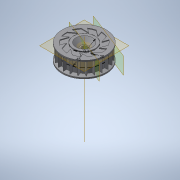
# Autodesk Inventor part: rear-wheel
Saved by Autodesk Inventor 2020 (Build 240168000, 168)
## iProperties
Created: 2020-01-27
Part Number: rear-wheel
Material: Ogólne
Document SubType Name: Modeling
Designer: blep
Density: 1 g/cm^3
Appearance: Domyślne
Author: blep
Autodesk Inventor part; units mm, degrees
ref_plane "YZ Plane" through (0, 0, 0) normal (1, 0, 0) x (0, 1, 0)
ref_plane "XZ Plane" through (0, 0, 0) normal (0, 1, 0) x (-1, 0, 0)
ref_plane "XY Plane" through (0, 0, 0) normal (0, 0, 1) x (1, 0, 0)
sketch "Sketch1" plane through (0, 0, 0) normal (0, 0, 1) x (1, 0, 0)
  line L0 (0.8361, -0.5831) -> (0.755, -0.1219) projected
  line L1 (0.6595, -0.0924) -> (0.3327, -0.4279) projected
  arc A0 (0.755, -0.1219) -> (0.6595, -0.0924) centre (0, -2.4) ccw projected
  arc A1 (0.3327, -0.4279) -> (0.2337, -0.4137) centre (0, -2.4) ccw projected
  arc A2 (0.9258, -0.6272) -> (0.8361, -0.5831) centre (0, -2.4) ccw projected
  line L2 (1.3403, -0.4091) -> (0.9258, -0.6272) projected
  arc A3 (1.4221, -0.4667) -> (1.3403, -0.4091) centre (0, -2.4) ccw projected
  line L3 (1.3566, -0.9304) -> (1.4221, -0.4667) projected
  arc A4 (1.4283, -1.0001) -> (1.3566, -0.9304) centre (0, -2.4) ccw projected
  line L4 (1.8899, -0.9207) -> (1.4283, -1.0001) projected
  arc A5 (1.9499, -1.0007) -> (1.8899, -0.9207) centre (0, -2.4) ccw projected
  line L5 (1.7443, -1.4216) -> (1.9499, -1.0007) projected
  arc A6 (1.791, -1.51) -> (1.7443, -1.4216) centre (0, -2.4) ccw projected
  line L6 (2.2545, -1.5772) -> (1.791, -1.51) projected
  arc A7 (2.2869, -1.6718) -> (2.2545, -1.5772) centre (0, -2.4) ccw projected
  line L7 (1.9613, -2.0085) -> (2.2869, -1.6718) projected
  arc A8 (1.9784, -2.107) -> (1.9613, -2.0085) centre (0, -2.4) ccw projected
  line L8 (2.3985, -2.3141) -> (1.9784, -2.107) projected
  arc A9 (2.4, -2.4141) -> (2.3985, -2.3141) centre (0, -2.4) ccw projected
  line L9 (1.9863, -2.6337) -> (2.4, -2.4141) projected
  arc A10 (1.9721, -2.7327) -> (1.9863, -2.6337) centre (0, -2.4) ccw projected
  line L10 (2.3076, -3.0595) -> (1.9721, -2.7327) projected
  line L11 (1.8169, -3.2361) -> (2.2781, -3.155) projected
  arc A11 (2.2781, -3.155) -> (2.3076, -3.0595) centre (0, -2.4) ccw projected
  arc A12 (1.7728, -3.3258) -> (1.8169, -3.2361) centre (0, -2.4) ccw projected
  line L12 (1.9909, -3.7403) -> (1.7728, -3.3258) projected
  arc A13 (1.9333, -3.8221) -> (1.9909, -3.7403) centre (0, -2.4) ccw projected
  line L13 (1.4696, -3.7566) -> (1.9333, -3.8221) projected
  arc A14 (1.3999, -3.8283) -> (1.4696, -3.7566) centre (0, -2.4) ccw projected
  line L14 (1.4793, -4.2899) -> (1.3999, -3.8283) projected
  arc A15 (1.3993, -4.3499) -> (1.4793, -4.2899) centre (0, -2.4) ccw projected
  line L15 (0.9784, -4.1443) -> (1.3993, -4.3499) projected
  arc A16 (0.89, -4.191) -> (0.9784, -4.1443) centre (0, -2.4) ccw projected
  line L16 (0.8228, -4.6545) -> (0.89, -4.191) projected
  arc A17 (0.7282, -4.6869) -> (0.8228, -4.6545) centre (0, -2.4) ccw projected
  line L17 (0.3915, -4.3613) -> (0.7282, -4.6869) projected
  arc A18 (0.293, -4.3784) -> (0.3915, -4.3613) centre (0, -2.4) ccw projected
  line L18 (0.0859, -4.7985) -> (0.293, -4.3784) projected
  arc A19 (-0.0141, -4.8) -> (0.0859, -4.7985) centre (0, -2.4) ccw projected
  line L19 (-0.2337, -4.3863) -> (-0.0141, -4.8) projected
  arc A20 (-0.3327, -4.3721) -> (-0.2337, -4.3863) centre (0, -2.4) ccw projected
  line L20 (-0.6595, -4.7076) -> (-0.3327, -4.3721) projected
  arc A21 (-0.755, -4.6781) -> (-0.6595, -4.7076) centre (0, -2.4) ccw projected
  line L21 (-0.8361, -4.2169) -> (-0.755, -4.6781) projected
  arc A22 (-0.9258, -4.1728) -> (-0.8361, -4.2169) centre (0, -2.4) ccw projected
  line L22 (-1.3403, -4.3909) -> (-0.9258, -4.1728) projected
  arc A23 (-1.4221, -4.3333) -> (-1.3403, -4.3909) centre (0, -2.4) ccw projected
  line L23 (-1.3566, -3.8696) -> (-1.4221, -4.3333) projected
  arc A24 (-1.4283, -3.7999) -> (-1.3566, -3.8696) centre (0, -2.4) ccw projected
  line L24 (-1.8899, -3.8793) -> (-1.4283, -3.7999) projected
  arc A25 (-1.9499, -3.7993) -> (-1.8899, -3.8793) centre (0, -2.4) ccw projected
  line L25 (-1.7443, -3.3784) -> (-1.9499, -3.7993) projected
  arc A26 (-1.791, -3.29) -> (-1.7443, -3.3784) centre (0, -2.4) ccw projected
  line L26 (-2.2545, -3.2228) -> (-1.791, -3.29) projected
  arc A27 (-2.2869, -3.1282) -> (-2.2545, -3.2228) centre (0, -2.4) ccw projected
  line L27 (-1.9613, -2.7915) -> (-2.2869, -3.1282) projected
  arc A28 (-1.9784, -2.693) -> (-1.9613, -2.7915) centre (0, -2.4) ccw projected
  line L28 (-2.3985, -2.4859) -> (-1.9784, -2.693) projected
  arc A29 (-2.4, -2.3859) -> (-2.3985, -2.4859) centre (0, -2.4) ccw projected
  line L29 (-1.9863, -2.1663) -> (-2.4, -2.3859) projected
  arc A30 (-1.9721, -2.0673) -> (-1.9863, -2.1663) centre (0, -2.4) ccw projected
  line L30 (-2.3076, -1.7405) -> (-1.9721, -2.0673) projected
  arc A31 (-2.2781, -1.645) -> (-2.3076, -1.7405) centre (0, -2.4) ccw projected
  line L31 (-1.8169, -1.5639) -> (-2.2781, -1.645) projected
  arc A32 (-1.7728, -1.4742) -> (-1.8169, -1.5639) centre (0, -2.4) ccw projected
  line L32 (-1.9909, -1.0597) -> (-1.7728, -1.4742) projected
  arc A33 (-1.9333, -0.9779) -> (-1.9909, -1.0597) centre (0, -2.4) ccw projected
  line L33 (-1.4696, -1.0434) -> (-1.9333, -0.9779) projected
  arc A34 (-1.3999, -0.9717) -> (-1.4696, -1.0434) centre (0, -2.4) ccw projected
  line L34 (-1.4793, -0.5101) -> (-1.3999, -0.9717) projected
  arc A35 (-1.3993, -0.4501) -> (-1.4793, -0.5101) centre (0, -2.4) ccw projected
  line L35 (-0.9784, -0.6557) -> (-1.3993, -0.4501) projected
  arc A36 (-0.89, -0.609) -> (-0.9784, -0.6557) centre (0, -2.4) ccw projected
  line L36 (-0.8228, -0.1455) -> (-0.89, -0.609) projected
  arc A37 (-0.7282, -0.1131) -> (-0.8228, -0.1455) centre (0, -2.4) ccw projected
  line L37 (-0.3915, -0.4387) -> (-0.7282, -0.1131) projected
  arc A38 (-0.293, -0.4216) -> (-0.3915, -0.4387) centre (0, -2.4) ccw projected
  line L38 (-0.0859, -0.0015) -> (-0.293, -0.4216) projected
  arc A39 (0.0141, 0) -> (-0.0859, -0.0015) centre (0, -2.4) ccw projected
  line L39 (0.2337, -0.4137) -> (0.0141, 0) projected
  line L40 (-0.4177, 0.0039) -> (-0.6435, 0.2222)
  arc A40 (-0.6435, 0.2222) -> (-1.095, 0.068) centre (0, -2.4) ccw
  line L41 (-1.095, 0.068) -> (-1.1401, -0.2428)
  line L42 (-1.1401, -0.2428) -> (-1.4223, -0.105)
  arc A41 (-1.4223, -0.105) -> (-1.8041, -0.3912) centre (0, -2.4) ccw
  line L43 (-1.8041, -0.3912) -> (-1.7509, -0.7007)
  line L44 (-1.7509, -0.7007) -> (-2.0619, -0.6568)
  arc A42 (-2.0619, -0.6568) -> (-2.3365, -1.047) centre (0, -2.4) ccw
  line L45 (-2.3365, -1.047) -> (-2.1903, -1.3249)
  line L46 (-2.1903, -1.3249) -> (-2.4996, -1.3793)
  arc A43 (-2.4996, -1.3793) -> (-2.6403, -1.8353) centre (0, -2.4) ccw
  line L47 (-2.6403, -1.8353) -> (-2.4153, -2.0544)
  line L48 (-2.4153, -2.0544) -> (-2.6927, -2.2017)
  arc A44 (-2.6927, -2.2017) -> (-2.6856, -2.6788) centre (0, -2.4) ccw
  line L49 (-2.6856, -2.6788) -> (-2.4039, -2.8177)
  line L50 (-2.4039, -2.8177) -> (-2.6222, -3.0435)
  arc A45 (-2.6222, -3.0435) -> (-2.468, -3.495) centre (0, -2.4) ccw
  line L51 (-2.468, -3.495) -> (-2.1572, -3.5401)
  line L52 (-2.1572, -3.5401) -> (-2.295, -3.8223)
  arc A46 (-2.295, -3.8223) -> (-2.0088, -4.2041) centre (0, -2.4) ccw
  line L53 (-2.0088, -4.2041) -> (-1.6993, -4.1509)
  line L54 (-1.6993, -4.1509) -> (-1.7432, -4.4619)
  arc A47 (-1.7432, -4.4619) -> (-1.353, -4.7365) centre (0, -2.4) ccw
  line L55 (-1.353, -4.7365) -> (-1.0751, -4.5903)
  line L56 (-1.0751, -4.5903) -> (-1.0207, -4.8996)
  arc A48 (-1.0207, -4.8996) -> (-0.5647, -5.0403) centre (0, -2.4) ccw
  line L57 (-0.5647, -5.0403) -> (-0.3456, -4.8153)
  line L58 (-0.3456, -4.8153) -> (-0.1983, -5.0927)
  arc A49 (-0.1983, -5.0927) -> (0.2788, -5.0856) centre (0, -2.4) ccw
  line L59 (0.2788, -5.0856) -> (0.4177, -4.8039)
  line L60 (0.4177, -4.8039) -> (0.6435, -5.0222)
  arc A50 (0.6435, -5.0222) -> (1.095, -4.868) centre (0, -2.4) ccw
  line L61 (1.095, -4.868) -> (1.1401, -4.5572)
  line L62 (1.1401, -4.5572) -> (1.4223, -4.695)
  arc A51 (1.4223, -4.695) -> (1.8041, -4.4088) centre (0, -2.4) ccw
  line L63 (1.8041, -4.4088) -> (1.7509, -4.0993)
  line L64 (1.7509, -4.0993) -> (2.0619, -4.1432)
  arc A52 (2.0619, -4.1432) -> (2.3365, -3.753) centre (0, -2.4) ccw
  line L65 (2.3365, -3.753) -> (2.1903, -3.4751)
  line L66 (2.1903, -3.4751) -> (2.4996, -3.4207)
  arc A53 (2.4996, -3.4207) -> (2.6403, -2.9647) centre (0, -2.4) ccw
  line L67 (2.6403, -2.9647) -> (2.4153, -2.7456)
  line L68 (2.4153, -2.7456) -> (2.6927, -2.5983)
  arc A54 (2.6927, -2.5983) -> (2.6856, -2.1212) centre (0, -2.4) ccw
  line L69 (2.6856, -2.1212) -> (2.4039, -1.9823)
  line L70 (2.4039, -1.9823) -> (2.6222, -1.7565)
  arc A55 (2.6222, -1.7565) -> (2.468, -1.305) centre (0, -2.4) ccw
  line L71 (2.468, -1.305) -> (2.1572, -1.2599)
  line L72 (2.1572, -1.2599) -> (2.295, -0.9777)
  arc A56 (2.295, -0.9777) -> (2.0088, -0.5959) centre (0, -2.4) ccw
  line L73 (2.0088, -0.5959) -> (1.6993, -0.6491)
  line L74 (1.6993, -0.6491) -> (1.7432, -0.3381)
  arc A57 (1.7432, -0.3381) -> (1.353, -0.0635) centre (0, -2.4) ccw
  line L75 (1.353, -0.0635) -> (1.0751, -0.2097)
  line L76 (1.0751, -0.2097) -> (1.0207, 0.0996)
  arc A58 (1.0207, 0.0996) -> (0.5647, 0.2403) centre (0, -2.4) ccw
  line L77 (0.5647, 0.2403) -> (0.3456, 0.0153)
  line L78 (0.3456, 0.0153) -> (0.1983, 0.2927)
  arc A59 (0.1983, 0.2927) -> (-0.2788, 0.2856) centre (0, -2.4) ccw
  line L79 (-0.2788, 0.2856) -> (-0.4177, 0.0039)
  circle A60 centre (0, -2.4) radius 22.5
  circle A61 centre (0, -2.4) radius 10
  point P0 (0, 0)
  dimension "d0" = 0.3
  dimension "d1" = 45
  dimension "d2" = 20
  constraints: 80 end point, 40 point on circle, 22 centre point, 2 coincident, 59 other
  measures "d0" distance between parallel lines of L38 L79
  measures "d1" diameter of A60
  measures "d2" diameter of A61
extrude "Extrusion1" add sketch "Sketch1" along normal blind 10.5 and the other way blind 9 contours A60
ref_plane "Work Plane3" through (0, -2.4, 0) normal (0.365, 0.931, 0) x (-0.931, 0.365, 0)
ref_plane "Work Plane2" through (8.212, 18.5479, 0) normal (0.365, 0.931, 0) x (-0.931, 0.365, 0)
sketch "Sketch2" plane through (0, -2.4, 0) normal (0.365, 0.931, 0) x (-0.931, 0.365, 0)
  line L0 (-22.5, -9) -> (-22.5, 10.5) projected
  line L1 (-22.5, -9) -> (22.5, -9) projected
  line L2 (22.5, 10.5) -> (-22.5, 10.5) projected
  line L3 (-22.5, -9) -> (-26.5, -9)
  line L4 (-26.5, -9) -> (-26.5, -7.5)
  line L5 (-22.5, 10.5) -> (-26.5, 10.5)
  line L6 (-26.5, 10.5) -> (-26.5, 9)
  line L7 (22.5, -9) -> (22.5, 10.5) projected
  line L8 (0, 10.5) -> (0, 40.5) construction
  line L9 (-26.5, 9) -> (-22.5, 7.5)
  line L10 (-26.5, -7.5) -> (-22.5, -6)
  line L11 (-22.5, 10.5) -> (-22.5, 7.5)
  line L12 (-22.5, -9) -> (-22.5, 10.5) projected
  line L13 (-22.5, -6) -> (-22.5, -9)
  point P0 (0.8759, 0)
  dimension "d7" = 1.5
  dimension "d8" = 1.5
  dimension "d9" = 4
  dimension "d73" = 3
  dimension "d74" = 3
  dimension "d77" = 30
  constraints: 18 end point, 3 perpendicular, 2 horizontal, 1 collinear, 1 midpoint, 1 point on line, 1 vertical
  measures "d7" distance of L3.end L4.end
  measures "d8" distance of L5.end L6.end
  measures "d9" distance between parallel lines of L0 L6
  measures "d73" distance of L0.end L9.end
  measures "d74" distance of L10.end L0.start
  measures "d77" distance from line of L8.end L2
revolve "Revolution1" add sketch "Sketch2" angle 360 about axis through (0, -2.4, 10.5) along (0, 0, 1) contours L3 L4 L10 L0 | L9 L6 L5 L0
sketch "Sketch3" plane through (0, -2.4, 10.5) normal (0, 0, 1) x (1, 0, 0)
  circle A0 centre (0, 0) radius 22.5 projected
  circle A1 centre (0, 0) radius 22.5 projected
  circle A2 centre (0, 0) radius 22.5 projected
  circle A3 centre (0, 0) radius 26.5 projected
  line L0 (0, 0) -> (0, -33.3322) construction
  line L1 (0, -25.5) -> (1.25, -22.4653)
  line L2 (0, -25.5) -> (-1.25, -22.4653)
  line L3 (1.7164, -22.5) -> (-4.3714, -22.5) construction
  line L4 (-1.25, -22.4653) -> (1.25, -22.4653)
  point P0 (0, 2.4)
  dimension "d14" = 3
  dimension "d15" = 1.25
  dimension "d16" = 1.25
  constraints: 12 end point, 2 point on circle, 1 horizontal, 1 perpendicular, 1 point on line, 1 tangent, 1 vertical
  measures "d14" distance from line of L1.start L3
  measures "d15" distance from line of L2.end L0
  measures "d16" distance from line of L0 L1.end
ref_plane "Work Plane4" through (0, -2.4, 7) normal (0, 0, 1) x (1, 0, 0)
extrude "Extrusion8" add sketch "Sketch3" against normal up to surface (19.5 mm away) contours A0 L1 L2
pattern_circular "Circular Pattern3" count 22 over 360 about axis through (0, -2.4, 10.5) along (0, 0, -1) of "Extrusion8"
sketch "Sketch6" plane through (0, -2.4, 10.5) normal (0, 0, 1) x (1, 0, 0)
  arc A0 (2.4996, -1.0207) -> (2.6403, -0.5647) centre (0, 0) ccw projected
  line L0 (2.6856, 0.2788) -> (2.4039, 0.4177) projected
  arc A1 (2.6927, -0.1983) -> (2.6856, 0.2788) centre (0, 0) ccw projected
  line L1 (2.4153, -0.3456) -> (2.6927, -0.1983) projected
  line L2 (2.6403, -0.5647) -> (2.4153, -0.3456) projected
  line L3 (2.1903, -1.0751) -> (2.4996, -1.0207) projected
  line L4 (2.3365, -1.353) -> (2.1903, -1.0751) projected
  arc A2 (2.0619, -1.7432) -> (2.3365, -1.353) centre (0, 0) ccw projected
  line L5 (1.7509, -1.6993) -> (2.0619, -1.7432) projected
  line L6 (1.8041, -2.0088) -> (1.7509, -1.6993) projected
  arc A3 (1.4223, -2.295) -> (1.8041, -2.0088) centre (0, 0) ccw projected
  line L7 (1.1401, -2.1572) -> (1.4223, -2.295) projected
  line L8 (1.095, -2.468) -> (1.1401, -2.1572) projected
  arc A4 (0.6435, -2.6222) -> (1.095, -2.468) centre (0, 0) ccw projected
  line L9 (0.4177, -2.4039) -> (0.6435, -2.6222) projected
  line L10 (0.2788, -2.6856) -> (0.4177, -2.4039) projected
  arc A5 (-0.1983, -2.6927) -> (0.2788, -2.6856) centre (0, 0) ccw projected
  line L11 (-0.3456, -2.4153) -> (-0.1983, -2.6927) projected
  line L12 (-0.5647, -2.6403) -> (-0.3456, -2.4153) projected
  arc A6 (-1.0207, -2.4996) -> (-0.5647, -2.6403) centre (0, 0) ccw projected
  line L13 (-1.0751, -2.1903) -> (-1.0207, -2.4996) projected
  line L14 (-1.353, -2.3365) -> (-1.0751, -2.1903) projected
  arc A7 (-1.7432, -2.0619) -> (-1.353, -2.3365) centre (0, 0) ccw projected
  line L15 (-1.6993, -1.7509) -> (-1.7432, -2.0619) projected
  line L16 (-2.0088, -1.8041) -> (-1.6993, -1.7509) projected
  arc A8 (-2.295, -1.4223) -> (-2.0088, -1.8041) centre (0, 0) ccw projected
  line L17 (-2.1572, -1.1401) -> (-2.295, -1.4223) projected
  line L18 (-2.468, -1.095) -> (-2.1572, -1.1401) projected
  arc A9 (-2.6222, -0.6435) -> (-2.468, -1.095) centre (0, 0) ccw projected
  line L19 (-2.4039, -0.4177) -> (-2.6222, -0.6435) projected
  line L20 (-2.6856, -0.2788) -> (-2.4039, -0.4177) projected
  arc A10 (-2.6927, 0.1983) -> (-2.6856, -0.2788) centre (0, 0) ccw projected
  line L21 (-2.4153, 0.3456) -> (-2.6927, 0.1983) projected
  line L22 (-2.6403, 0.5647) -> (-2.4153, 0.3456) projected
  arc A11 (-2.4996, 1.0207) -> (-2.6403, 0.5647) centre (0, 0) ccw projected
  line L23 (-2.1903, 1.0751) -> (-2.4996, 1.0207) projected
  line L24 (-2.3365, 1.353) -> (-2.1903, 1.0751) projected
  arc A12 (-2.0619, 1.7432) -> (-2.3365, 1.353) centre (0, 0) ccw projected
  line L25 (-1.7509, 1.6993) -> (-2.0619, 1.7432) projected
  line L26 (-1.8041, 2.0088) -> (-1.7509, 1.6993) projected
  arc A13 (-1.4223, 2.295) -> (-1.8041, 2.0088) centre (0, 0) ccw projected
  line L27 (-1.1401, 2.1572) -> (-1.4223, 2.295) projected
  line L28 (-1.095, 2.468) -> (-1.1401, 2.1572) projected
  arc A14 (-0.6435, 2.6222) -> (-1.095, 2.468) centre (0, 0) ccw projected
  line L29 (-0.4177, 2.4039) -> (-0.6435, 2.6222) projected
  line L30 (-0.2788, 2.6856) -> (-0.4177, 2.4039) projected
  arc A15 (0.1983, 2.6927) -> (-0.2788, 2.6856) centre (0, 0) ccw projected
  line L31 (0.3456, 2.4153) -> (0.1983, 2.6927) projected
  line L32 (0.5647, 2.6403) -> (0.3456, 2.4153) projected
  arc A16 (1.0207, 2.4996) -> (0.5647, 2.6403) centre (0, 0) ccw projected
  line L33 (1.0751, 2.1903) -> (1.0207, 2.4996) projected
  line L34 (1.353, 2.3365) -> (1.0751, 2.1903) projected
  arc A17 (1.7432, 2.0619) -> (1.353, 2.3365) centre (0, 0) ccw projected
  line L35 (1.6993, 1.7509) -> (1.7432, 2.0619) projected
  line L36 (2.0088, 1.8041) -> (1.6993, 1.7509) projected
  arc A18 (2.295, 1.4223) -> (2.0088, 1.8041) centre (0, 0) ccw projected
  line L37 (2.1572, 1.1401) -> (2.295, 1.4223) projected
  line L38 (2.468, 1.095) -> (2.1572, 1.1401) projected
  arc A19 (2.6222, 0.6435) -> (2.468, 1.095) centre (0, 0) ccw projected
  line L39 (2.4039, 0.4177) -> (2.6222, 0.6435) projected
  circle A20 centre (0, 0) radius 10 projected
  point P0 (0, 2.4)
extrude "Extrusion4" add sketch "Sketch6" against normal blind 14.5 contours L3 L4 A2 L5 L6 A3 L7 L8 A4 L9 L10 A5 L11 L12 A6 L13 L14 A7 L15 L16 A8 L17 L18 A9 L19 L20 A10 L21 L22 A11 L23 L24 A12 L25 L26 A13 L27 L28 A14 L29 L30 A15 L31 L32 A16 L33 L34 A17 L35 L36 A18 L37 L38 A19 L39 L0 A1 L1 L2 A0 | A20
extrude "Extrusion5" cut sketch "Sketch6" against normal blind 9.5 contours L3 L4 A2 L5 L6 A3 L7 L8 A4 L9 L10 A5 L11 L12 A6 L13 L14 A7 L15 L16 A8 L17 L18 A9 L19 L20 A10 L21 L22 A11 L23 L24 A12 L25 L26 A13 L27 L28 A14 L29 L30 A15 L31 L32 A16 L33 L34 A17 L35 L36 A18 L37 L38 A19 L39 L0 A1 L1 L2 A0 | A20
sketch "Sketch7" plane through (0, -2.4, 1) normal (0, 0, 1) x (1, 0, 0)
  circle A0 centre (0, 0) radius 10 projected
  circle A1 centre (0, 0) radius 3
  point P0 (0, 2.4)
  dimension "d30" = 6
  constraints: 1 centre point, 1 coincident
  measures "d30" diameter of A1
extrude "Extrusion6" add sketch "Sketch7" along normal blind 4
sketch "Sketch8" plane through (0, -2.4, 10.5) normal (0, 0, 1) x (1, 0, 0)
  circle A0 centre (0, -1.5) radius 1.25
  circle A1 centre (0, -1.5) radius 22
  circle A2 centre (0, -1.5) radius 14.5
  circle A3 centre (0, 0) radius 26.5 projected
  circle A4 centre (0, 0) radius 10 projected
  line L0 (-16.5454, 13) -> (0, 13)
  line L1 (-12.2839, 13) -> (8.7765, 13) construction
  line L2 (0, 0) -> (0, 34.5807) construction
  line L3 (-20.6821, 6) -> (-12.4097, 6)
  point P0 (0, 2.4)
  dimension "d34" = 3
  dimension "d36" = 3
  dimension "d37" = 90
  dimension "d38" = 7
  dimension "d61" = 44
  dimension "d62" = 2.5
  dimension "d63" = 8.7765
  dimension "d65" = 12.2839
  constraints: 8 end point, 4 point on circle, 3 centre point, 2 coincident, 2 tangent, 1 parallel, 1 perpendicular, 1 point on line, 1 vertical
  measures "d37" angle of L2 L0
  measures "d38" distance between parallel lines of L3 L0
  measures "d61" diameter of A1
  measures "d62" diameter of A0
  measures "d63" distance from line of L1.end L2
  measures "d65" distance from line of L1.start L2
extrude "Extrusion7" cut sketch "Sketch8" against normal blind 1 contours L0 A2 L3 A1 picked at (-13.7464, 8.4059)
pattern_circular "Circular Pattern2" count 10 over 360 about axis through (0, -2.4, 10.5) along (0, 0, -1) of "Extrusion7"
chamfer "Chamfer1" distance 5.5 distance2 5.5 1 edges at (-10, -2.4, 5) measured on face at (9.8705, -4.0041, 8.6667)
sketch "Sketch12" plane through (0, -2.4, -9) normal (0, 0, -1) x (-1, 0, 0)
  circle A0 centre (0, 0) radius 10 projected
  point P0 (0, 2.4)
extrude "Extrusion12" cut sketch "Sketch12" against normal blind 10
ref_plane "Work Plane1" through (23.8056, -18.3916, -47.4) normal (0.365, 0.931, 0) x (0.931, -0.365, 0)
equation "\"d16\" = d15"
equation "\"d36\" = d34"
equation "\"d7\" = d8"
equation "\"d74\" = d73"
body "Solid1"
